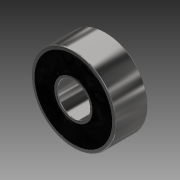
# Autodesk Inventor part: fc18-073
Saved by Autodesk Inventor 2018 (Build 220112000, 112)
## iProperties
Category: Bearing
Company: Autodesk Inc.
Created: 2017-11-24
Part Number: fc18-073
Material: Stainless Steel, 440C
Document SubType Name: Modeling
Designer: Autodesk Inc.
Density: 7.75 g/cm^3
Appearance: Steel - Polished
Catalog Web Link: http://www.shusterbearings.com/shopexd.asp?id=98
Vendor: Shuster
Author: Autodesk Inc.
Keywords: FIRST Choice
Autodesk Inventor part; units mm, degrees
ref_plane "YZ Plane" through (0, 0, 0) normal (1, 0, 0) x (0, 1, 0)
ref_plane "XZ Plane" through (0, 0, 0) normal (0, 1, 0) x (-1, 0, 0)
sketch "Sketch1" plane through (0, 0, 0) normal (0, 1, 0) x (-1, 0, 0)
  circle A0 centre (0, 0) radius 5
  circle A1 centre (0, 0) radius 13
  dimension "d0" = 10
  dimension "d1" = 26
  constraints: 2 centre point, 2 coincident
  measures "d0" diameter of A0
  measures "d1" diameter of A1
extrude "Extrusion1" add sketch "Sketch1" against normal blind 10
fillet "Fillet1" radius 0.3 4 edges at (13, 0, 0) (13, -10, 0) (5, 0, 0) (5, -10, 0)
sketch "Sketch2" plane through (0, 0, 0) normal (1, 0, 0) x (0, 1, 0)
  line L0 (-10, -12.7) -> (-10, 12.7) projected
  line L1 (-0.3, 13) -> (-9.7, 13) projected
  line L2 (-12.3802, 0) -> (2.0634, 0) projected
  circle A0 centre (-10, 11.688) radius 0.25
  circle A1 centre (-10, 6.137) radius 0.25
  point P0 (0, 0)
  dimension "d6" = 0.5
  constraints: 2 centre point, 2 point on line, 1 equal radius
  measures "d6" diameter of A0
revolve "Revolution1" cut sketch "Sketch2" angle 360 about axis through (0, -10, 0) along (0, 1, 0)
ref_plane "Work Plane2" through (0, -5, 0) normal (0, -1, 0) x (1, 0, 0)
mirror "Mirror2" about plane through (0, -5, 0) normal (0, -1, 0) of "Revolution1"
body "Solid1"
